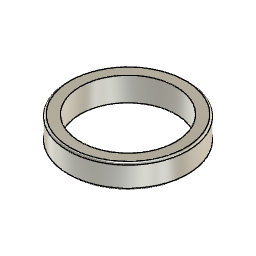
Cesaroni 29Pro 2G regular closure v3 (Autodesk Fusion 360 design; units mm, degrees)
Autodesk Fusion 360 part; units mm, degrees
sketch "Sketch1" plane through (0, 0, 0) normal (0, 0, 1) x (1, 0, 0)
  circle A0 centre (0, 0) radius 15.875
  circle A1 centre (0, 0) radius 12.7
  dimension "d1" = 31.75
  dimension "d2" = 25.4
  constraint coincident A0.centre A1.centre
  constraint concentric A0 A1
  measures "d1" diameter of A0
  measures "d2" diameter of A1
extrude "Extrude1" add sketch "Sketch1" along normal blind 6.35
fillet "Fillet1" radius 0.5 2 edges at (-14.8007, -5.7406, 0) (-14.8007, -5.7406, 6.35)
